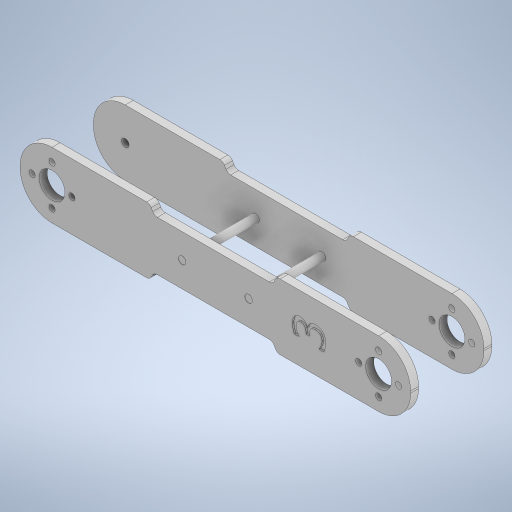
# Autodesk Inventor part: Pieza_eslabon_3
Saved by Autodesk Inventor 2023 (Build 270158000, 158)
## iProperties
Created: 2024-09-21
Part Number: Pieza_eslabon_3
Material: Genérico
Document SubType Name: Sheet Metal
Designer: sebas
Density: 1 g/cm^3
Sheet Metal Rule: Por defecto_mm
Appearance: Valor por defecto
Author: sebas
Autodesk Inventor part; units mm, degrees
ref_plane "YZ Plane" through (0, 0, 0) normal (1, 0, 0) x (0, 1, 0)
ref_plane "XZ Plane" through (0, 0, 0) normal (0, 1, 0) x (-1, 0, 0)
sketch "Boceto1" plane through (0, 0, 0) normal (0, 0, 1) x (1, 0, 0)
  line L0 (-73.5, -0.35) -> (-73.5, 0.35)
  line L1 (73.5, 0.35) -> (73.5, -0.35)
  line L2 (73.5, -12.35) -> (-73.5, 12.35) construction
  line L3 (-73.5, -12.35) -> (73.5, 12.35) construction
  arc A0 (-61.5, 12.35) -> (-73.5, 0.35) centre (-61.5, 0.35) ccw
  arc A1 (-73.5, -0.35) -> (-61.5, -12.35) centre (-61.5, -0.35) ccw
  arc A2 (61.5, -12.35) -> (73.5, -0.35) centre (61.5, -0.35) ccw
  arc A3 (73.5, 0.35) -> (61.5, 12.35) centre (61.5, 0.35) ccw
  line L4 (-21.8453, 9.35) -> (20.3453, 9.35)
  line L5 (22.0774, 10.35) -> (22.6547, 11.35)
  line L6 (-23.5774, 10.35) -> (-24.1547, 11.35)
  line L7 (-61.5, 12.35) -> (-25.8868, 12.35)
  line L8 (24.3868, 12.35) -> (61.5, 12.35)
  line L9 (0, 0) -> (44.6229, 0) construction
  line L10 (-21.8453, -9.35) -> (20.3453, -9.35)
  line L11 (22.0774, -10.35) -> (22.6547, -11.35)
  line L12 (-23.5774, -10.35) -> (-24.1547, -11.35)
  line L13 (61.5, -12.35) -> (24.3868, -12.35)
  line L14 (-25.8868, -12.35) -> (-61.5, -12.35)
  arc A4 (-24.1547, 11.35) -> (-25.8868, 12.35) centre (-25.8868, 10.35) ccw
  arc A5 (-23.5774, 10.35) -> (-21.8453, 9.35) centre (-21.8453, 11.35) ccw
  arc A6 (20.3453, 9.35) -> (22.0774, 10.35) centre (20.3453, 11.35) ccw
  arc A7 (24.3868, 12.35) -> (22.6547, 11.35) centre (24.3868, 10.35) ccw
  arc A8 (22.6547, -11.35) -> (24.3868, -12.35) centre (24.3868, -10.35) ccw
  arc A9 (22.0774, -10.35) -> (20.3453, -9.35) centre (20.3453, -11.35) ccw
  arc A10 (-21.8453, -9.35) -> (-23.5774, -10.35) centre (-21.8453, -11.35) ccw
  arc A11 (-25.8868, -12.35) -> (-24.1547, -11.35) centre (-25.8868, -10.35) ccw
  point P0 (-23, 9.35)
  point P1 (21.5, 9.35)
  point P2 (73.5, 0)
  point P3 (23.2321, 12.35)
  point P4 (-24.7321, 12.35)
  point P5 (-23, -9.35)
  point P6 (21.5, -9.35)
  point P7 (23.2321, -12.35)
  point P8 (-24.7321, -12.35)
  dimension "d0" = 147
  dimension "d1" = 24.7
  dimension "d2" = 12
  dimension "d5" = 3
  dimension "d6" = 120
  dimension "d7" = 120
  dimension "d8" = 52
  dimension "d9" = 12
  dimension "d10" = 2
  dimension "d11" = 2
  constraints: 30 end point, 28 tangent, 24 point on circle, 20 point on line, 12 centre point, 9 equal radius, 5 parallel, 4 horizontal, 4 symmetric about line, 3 midpoint, 2 perpendicular
  measures "d0" distance of L2.end L3.end
  measures "d1" distance of L3.start L2.end
  measures "d2" radius of A0
  measures "d5" distance between parallel lines of L8 L4
  measures "d6" angle of L4 L5
  measures "d7" angle of L4 L6
  measures "d8" horizontal distance of L1.start point (21.5, 9.35)
  measures "d9" radius of A3
  measures "d10" radius of A4
  measures "d11" radius of A10
extrude "Extrusión1" add sketch "Boceto1" along normal mid plane 3
sketch "Boceto2" plane through (0, 0, 1.5) normal (0, 0, 1) x (1, 0, 0)
  arc A0 (73.5, 0.35) -> (61.5, 12.35) centre (61.5, 0.35) ccw construction
  circle A1 centre (61.5, 0) radius 7.5 construction
  circle A2 centre (61.5, 0) radius 4.85
  circle A3 centre (54, 0) radius 1.15
  circle A4 centre (61.5, 0) radius 7.5 construction
  circle A5 centre (61.5, -7.5) radius 1.15
  circle A6 centre (61.5, 0) radius 7.5 construction
  circle A7 centre (69, 0) radius 1.15
  circle A8 centre (61.5, 0) radius 7.5 construction
  circle A9 centre (61.5, 7.5) radius 1.15
  point P0 (0, 0)
  dimension "d14" = 15
  dimension "d15" = 9.7
  dimension "d16" = 2.3
  dimension "d19" = 360
  constraints: 5 centre point, 3 coincident, 2 horizontal alignment, 2 vertical alignment, 23 other
  measures "d15" diameter of A2
  measures "d16" diameter of A3
extrude "Extrusión2" cut sketch "Boceto2" against normal up to surface (3 mm away)
sketch "Boceto3" plane through (0, 0, 1.5) normal (0, 0, 1) x (1, 0, 0)
  arc A0 (-61.5, 12.35) -> (-73.5, 0.35) centre (-61.5, 0.35) ccw construction
  circle A1 centre (-12.5, 0) radius 1.4
  circle A2 centre (12.5, 0) radius 1.4
  line L0 (0, 0) -> (0, 9) construction
  dimension "d24" = 2.8
  dimension "d25" = 2.8
  dimension "d26" = 25
  dimension "d27" = 12.5
  constraints: 2 centre point, 2 end point
  measures "d24" diameter of A1
  measures "d25" diameter of A2
  measures "d26" distance of A2.centre A1.centre
  measures "d27" distance from line of A2.centre L0
extrude "Extrusión3" cut sketch "Boceto3" against normal up to surface (3 mm away)
ref_plane "Plano de trabajo1" through (0, 0, 13.8) normal (0, 0, 1) x (1, 0, 0)
mirror "Simetría1" about plane through (0, 0, 13.8) normal (0, 0, 1) of "Extrusión1", "Extrusión2", "Extrusión3"
sketch "Boceto4" plane through (-21.8453, -9.35, 29.1) normal (0, 0, 1) x (1, 0, 0)
  line L0 (21.8453, 9.35) -> (21.8453, 51) construction
  circle A0 centre (83.3453, 9.35) radius 4.85 projected
  circle A1 centre (75.8453, 9.35) radius 1.15 projected
  circle A2 centre (83.3453, 16.85) radius 1.15 projected
  circle A3 centre (90.8453, 9.35) radius 1.15 projected
  circle A4 centre (83.3453, 1.85) radius 1.15 projected
  circle A5 centre (-39.6547, 9.35) radius 4.85
  circle A6 centre (-32.1547, 9.35) radius 1.15
  circle A7 centre (-39.6547, 16.85) radius 1.15
  circle A8 centre (-47.1547, 9.35) radius 1.15
  circle A9 centre (-39.6547, 1.85) radius 1.15
  constraints: 5 centre point, 5 symmetric about line, 2 end point, 1 vertical, 5 other
extrude "Extrusión4" cut sketch "Boceto4" against normal up to surface (3 mm away) contours A5 | A6 | A7 | A8 | A9
sketch "Boceto5" plane through (0, 0, -1.5) normal (0, 0, -1) x (-1, 0, 0)
  arc A0 (73.5, 0.35) -> (61.5, 12.35) centre (61.5, 0.35) ccw construction
  circle A1 centre (61.5, 0) radius 1.4
  point P0 (0, 0)
  dimension "d33" = 2.8
  constraints: 1 centre point
  measures "d33" diameter of A1
extrude "Extrusión5" cut sketch "Boceto5" against normal up to surface (3 mm away)
sketch "Boceto6" plane through (0, 0, 13.8) normal (0, 0, 1) x (1, 0, 0)
  circle A0 centre (-12.5, 0) radius 1.4 projected
  circle A1 centre (12.5, 0) radius 1.4 projected
  point P0 (0, 0)
extrude "Extrusión6" add sketch "Boceto6" along normal mid plane 30.5
sketch "Boceto7" plane through (-21.8453, -9.35, 29.1) normal (0, 0, 1) x (1, 0, 0)
  line L0 (50.9088, 5.399) -> (50.9088, 24.6396) construction
  line L1 (50.9088, 24.6396) -> (65.6599, 24.6396) construction
  line L2 (65.6599, 24.6396) -> (65.6599, 5.399) construction
  line L3 (65.6599, 5.399) -> (50.9088, 5.399) construction
  spline S0 degree 2 poles (52.2994, 9.5125) (52.2994, 9.0749) (52.5133, 8.2094) (52.6786, 7.7912) knots 0 0 0 1 2 2 2
  spline S1 degree 2 poles (52.6786, 7.7912) (52.844, 7.4022) (53.194, 6.8285) (53.3496, 6.6048) knots 0 0 0 1 2 2 2
  line L4 (53.3496, 6.6048) -> (53.3496, 6.5076)
  line L5 (53.3496, 6.5076) -> (51.6479, 6.5076)
  spline S2 degree 2 poles (51.6479, 6.5076) (51.3658, 7.0327) (50.9088, 8.8317) (50.9088, 9.6389) knots 0 0 0 1 2 2 2
  spline S3 degree 2 poles (50.9088, 9.6389) (50.9088, 10.4557) (51.2394, 11.6713) (51.5895, 12.1672) knots 0 0 0 1 2 2 2
  spline S4 degree 2 poles (51.5895, 12.1672) (51.9688, 12.6924) (53.0676, 13.2369) (53.8067, 13.2369) knots 0 0 0 1 2 2 2
  spline S5 degree 2 poles (53.8067, 13.2369) (54.7986, 13.2369) (56.2962, 11.9339) (56.4906, 11.0197) knots 0 0 0 1 2 2 2
  line L6 (56.4906, 11.0197) -> (56.6073, 11.0197)
  spline S6 degree 2 poles (56.6073, 11.0197) (56.6851, 11.399) (57.0352, 12.2645) (57.3853, 12.634) knots 0 0 0 1 2 2 2
  spline S7 degree 2 poles (57.3853, 12.634) (57.7257, 13.0035) (58.8148, 13.4703) (59.6025, 13.4703) knots 0 0 0 1 2 2 2
  spline S8 degree 2 poles (59.6025, 13.4703) (60.4096, 13.4703) (61.7808, 12.916) (62.3059, 12.4103) knots 0 0 0 1 2 2 2
  spline S9 degree 2 poles (62.3059, 12.4103) (62.8504, 11.8852) (63.4145, 10.3974) (63.4145, 9.4541) knots 0 0 0 1 2 2 2
  spline S10 degree 2 poles (63.4145, 9.4541) (63.4145, 8.5497) (62.9769, 6.7799) (62.6754, 6.177) knots 0 0 0 1 2 2 2
  line L7 (62.6754, 6.177) -> (60.9736, 6.177)
  line L8 (60.9736, 6.177) -> (60.9736, 6.2937)
  spline S11 degree 2 poles (60.9736, 6.2937) (61.3432, 6.7993) (62.0239, 8.5108) (62.0239, 9.3569) knots 0 0 0 1 2 2 2
  spline S12 degree 2 poles (62.0239, 9.3569) (62.0239, 9.8528) (61.7127, 10.8447) (61.3529, 11.1753) knots 0 0 0 1 2 2 2
  spline S13 degree 2 poles (61.3529, 11.1753) (60.9931, 11.4962) (60.1373, 11.8366) (59.4858, 11.8366) knots 0 0 0 1 2 2 2
  spline S14 degree 2 poles (59.4858, 11.8366) (58.8342, 11.8366) (57.9882, 11.4574) (57.7451, 11.117) knots 0 0 0 1 2 2 2
  spline S15 degree 2 poles (57.7451, 11.117) (57.502, 10.7766) (57.3172, 9.8528) (57.3172, 9.3082) knots 0 0 0 1 2 2 2
  line L9 (57.3172, 9.3082) -> (57.3172, 8.6275)
  line L10 (57.3172, 8.6275) -> (55.985, 8.6275)
  line L11 (55.985, 8.6275) -> (55.985, 9.1624)
  spline S16 degree 2 poles (55.985, 9.1624) (55.985, 10.2418) (54.9542, 11.6032) (53.972, 11.6032) knots 0 0 0 1 2 2 2
  spline S17 degree 2 poles (53.972, 11.6032) (53.515, 11.6032) (52.8634, 11.2531) (52.6689, 10.9711) knots 0 0 0 1 2 2 2
  spline S18 degree 2 poles (52.6689, 10.9711) (52.4647, 10.6697) (52.2994, 9.9306) (52.2994, 9.5125) knots 0 0 0 1 2 2 2
  point P0 (21.8453, 9.35)
  constraints: 2 other
extrude "Extrusión7" cut sketch "Boceto7" against normal blind 0.5
equation "\"Radio_pliegue\" = Grosor"
equation "\"Anchura_desahogo_plegado\" = Grosor"
equation "\"Profundidad_desahogo_plegado\" = 0.5 * Grosor"
equation "\"Tamaño_destalonado\" = 4 * Grosor"
equation "\"Remanente_mínimo\" = 2 * Grosor"
equation "\"Radiodetransición\" = Radio_pliegue"
equation "\"Tamaño_de_radio_de_Jacobi\" = Radio_pliegue"
equation "\"TamañoSeparación\" = Grosor"
equation "\"Grosor\" = 0.5"
